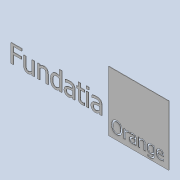
# Autodesk Inventor part: Orange
Saved by Autodesk Inventor 2020 (Build 240168000, 168)
## iProperties
Created: 2021-04-30
Part Number: Orange
Material: Generic
Document SubType Name: Modeling
Designer: Iulian Bors
Density: 1 g/cm^3
Appearance: Default
Author: Iulian Bors
Autodesk Inventor part; units mm, degrees
ref_plane "YZ Plane" through (0, 0, 0) normal (1, 0, 0) x (0, 1, 0)
ref_plane "XZ Plane" through (0, 0, 0) normal (0, 1, 0) x (-1, 0, 0)
ref_plane "XY Plane" through (0, 0, 0) normal (0, 0, 1) x (1, 0, 0)
sketch "Sketch1" plane through (0, 0, 0) normal (0, 0, 1) x (1, 0, 0)
  line L0 (-148.5, 210) -> (148.5, 210) construction
  line L1 (148.5, 210) -> (148.5, -210) construction
  line L2 (148.5, -210) -> (-148.5, -210) construction
  line L3 (-148.5, -210) -> (-148.5, 210) construction
  line L4 (22.4766, 60.7197) -> (122.4766, 60.7197)
  line L5 (122.4766, 60.7197) -> (122.4766, -39.2803)
  line L6 (122.4766, -39.2803) -> (22.4766, -39.2803)
  line L7 (22.4766, -39.2803) -> (22.4766, 60.7197)
  line L8 (26.6157, -0.7486) -> (40.1539, -0.7486) construction
  line L9 (40.1539, -0.7486) -> (40.1539, -4.7253) construction
  line L10 (40.1539, -4.7253) -> (26.6157, -4.7253) construction
  line L11 (26.6157, -4.7253) -> (26.6157, -0.7486) construction
  line L12 (-143.5348, 14.9841) -> (-38.9481, 14.9841) construction
  line L13 (-38.9481, 14.9841) -> (-38.9481, -7.7905) construction
  line L14 (-38.9481, -7.7905) -> (-143.5348, -7.7905) construction
  line L15 (-143.5348, -7.7905) -> (-143.5348, 14.9841) construction
  line L16 (-122.5543, 10.0975) -> (-136.5089, 10.0975)
  line L17 (-136.5089, 10.0975) -> (-136.5089, 1.6373)
  line L18 (-136.5089, 1.6373) -> (-123.1377, 1.6373)
  line L19 (-123.1377, 1.6373) -> (-123.1377, -1.9122)
  line L20 (-123.1377, -1.9122) -> (-136.5089, -1.9122)
  line L21 (-136.5089, -1.9122) -> (-136.5089, -16.353)
  line L22 (-136.5089, -16.353) -> (-140.4959, -16.353)
  line L23 (-140.4959, -16.353) -> (-140.4959, 13.647)
  line L24 (-140.4959, 13.647) -> (-122.5543, 13.647)
  line L25 (-122.5543, 13.647) -> (-122.5543, 10.0975)
  line L26 (-101.7682, -16.353) -> (-105.5608, -16.353)
  line L27 (-105.5608, -16.353) -> (-105.5608, -13.8733)
  spline S0 degree 2 poles (-105.5608, -13.8733) (-107.3112, -15.4049) (-110.4473, -16.9851) (-112.3922, -16.9851) knots 0 0 0 1 2 2 2
  spline S1 degree 2 poles (-112.3922, -16.9851) (-113.8509, -16.9851) (-116.4522, -16.0127) (-117.4003, -14.9673) knots 0 0 0 1 2 2 2
  spline S2 degree 2 poles (-117.4003, -14.9673) (-118.3728, -13.9219) (-119.4424, -10.7371) (-119.4424, -8.4519) knots 0 0 0 1 2 2 2
  line L28 (-119.4424, -8.4519) -> (-119.4424, 6.1591)
  line L29 (-119.4424, 6.1591) -> (-115.6499, 6.1591)
  line L30 (-115.6499, 6.1591) -> (-115.6499, -6.6772)
  spline S3 degree 2 poles (-115.6499, -6.6772) (-115.6499, -8.4762) (-115.3825, -10.8344) (-114.9206, -11.7096) knots 0 0 0 1 2 2 2
  spline S4 degree 2 poles (-114.9206, -11.7096) (-114.4587, -12.5848) (-112.8784, -13.3871) (-111.3954, -13.3871) knots 0 0 0 1 2 2 2
  spline S5 degree 2 poles (-111.3954, -13.3871) (-110.0097, -13.3871) (-106.8736, -11.8068) (-105.5608, -10.6642) knots 0 0 0 1 2 2 2
  line L31 (-105.5608, -10.6642) -> (-105.5608, 6.1591)
  line L32 (-105.5608, 6.1591) -> (-101.7682, 6.1591)
  line L33 (-101.7682, 6.1591) -> (-101.7682, -16.353)
  line L34 (-78.5997, -16.353) -> (-82.3922, -16.353)
  line L35 (-82.3922, -16.353) -> (-82.3922, -3.5167)
  spline S6 degree 2 poles (-82.3922, -3.5167) (-82.3922, -1.9608) (-82.6839, 0.7134) (-83.1215, 1.5157) knots 0 0 0 1 2 2 2
  spline S7 degree 2 poles (-83.1215, 1.5157) (-83.5835, 2.3666) (-85.2366, 3.1932) (-86.6467, 3.1932) knots 0 0 0 1 2 2 2
  spline S8 degree 2 poles (-86.6467, 3.1932) (-88.0567, 3.1932) (-91.047, 1.6859) (-92.4813, 0.4703) knots 0 0 0 1 2 2 2
  line L36 (-92.4813, 0.4703) -> (-92.4813, -16.353)
  line L37 (-92.4813, -16.353) -> (-96.2739, -16.353)
  line L38 (-96.2739, -16.353) -> (-96.2739, 6.1591)
  line L39 (-96.2739, 6.1591) -> (-92.4813, 6.1591)
  line L40 (-92.4813, 6.1591) -> (-92.4813, 3.6551)
  spline S9 degree 2 poles (-92.4813, 3.6551) (-90.7796, 5.1867) (-87.4976, 6.7912) (-85.6499, 6.7912) knots 0 0 0 1 2 2 2
  spline S10 degree 2 poles (-85.6499, 6.7912) (-82.3436, 6.7912) (-78.5997, 2.4152) (-78.5997, -1.742) knots 0 0 0 1 2 2 2
  line L41 (-78.5997, -1.742) -> (-78.5997, -16.353)
  line L42 (-55.9659, -16.353) -> (-59.7585, -16.353)
  line L43 (-59.7585, -16.353) -> (-59.7585, -14.0678)
  spline S11 degree 2 poles (-59.7585, -14.0678) (-60.6337, -14.7971) (-61.9222, -15.7696) (-62.7974, -16.1828) knots 0 0 0 1 2 2 2
  spline S12 degree 2 poles (-62.7974, -16.1828) (-63.5997, -16.5718) (-65.3258, -16.9851) (-66.4684, -16.9851) knots 0 0 0 1 2 2 2
  spline S13 degree 2 poles (-66.4684, -16.9851) (-68.316, -16.9851) (-71.4279, -15.4535) (-72.5219, -13.9705) knots 0 0 0 1 2 2 2
  spline S14 degree 2 poles (-72.5219, -13.9705) (-73.6159, -12.4875) (-74.8314, -8.1115) (-74.8314, -5.2671) knots 0 0 0 1 2 2 2
  spline S15 degree 2 poles (-74.8314, -5.2671) (-74.8314, -2.3012) (-73.2998, 2.0262) (-71.9627, 3.6551) knots 0 0 0 1 2 2 2
  spline S16 degree 2 poles (-71.9627, 3.6551) (-70.7228, 5.1138) (-67.2463, 6.7912) (-65.3258, 6.7912) knots 0 0 0 1 2 2 2
  spline S17 degree 2 poles (-65.3258, 6.7912) (-63.6483, 6.7912) (-61.1442, 6.0376) (-59.7585, 5.2596) knots 0 0 0 1 2 2 2
  line L44 (-59.7585, 5.2596) -> (-59.7585, 14.9841)
  line L45 (-59.7585, 14.9841) -> (-55.9659, 14.9841)
  line L46 (-55.9659, 14.9841) -> (-55.9659, -16.353)
  line L47 (-59.7585, -10.883) -> (-59.7585, 2.1235)
  spline S18 degree 2 poles (-59.7585, 2.1235) (-61.1685, 2.8042) (-63.4052, 3.3147) (-64.6937, 3.3147) knots 0 0 0 1 2 2 2
  spline S19 degree 2 poles (-64.6937, 3.3147) (-67.611, 3.3147) (-70.9173, -1.0613) (-70.9173, -5.1942) knots 0 0 0 1 2 2 2
  spline S20 degree 2 poles (-70.9173, -5.1942) (-70.9173, -9.1812) (-68.389, -13.3871) (-65.5932, -13.3871) knots 0 0 0 1 2 2 2
  spline S21 degree 2 poles (-65.5932, -13.3871) (-64.1102, -13.3871) (-61.0956, -12.0256) (-59.7585, -10.883) knots 0 0 0 1 2 2 2
  spline S22 degree 2 poles (-37.927, -13.9705) (-38.389, -14.3109) (-39.9449, -15.5264) (-40.6742, -15.8911) knots 0 0 0 1 2 2 2
  spline S23 degree 2 poles (-40.6742, -15.8911) (-41.671, -16.426) (-43.5429, -16.9851) (-45.2447, -16.9851) knots 0 0 0 1 2 2 2
  spline S24 degree 2 poles (-45.2447, -16.9851) (-46.6305, -16.9851) (-49.1345, -15.9397) (-50.0826, -14.9916) knots 0 0 0 1 2 2 2
  spline S25 degree 2 poles (-50.0826, -14.9916) (-50.9822, -14.0678) (-52.0762, -11.3449) (-52.0762, -9.8376) knots 0 0 0 1 2 2 2
  spline S26 degree 2 poles (-52.0762, -9.8376) (-52.0762, -7.5038) (-50.107, -4.1974) (-47.9676, -3.2493) knots 0 0 0 1 2 2 2
  spline S27 degree 2 poles (-47.9676, -3.2493) (-46.0713, -2.3741) (-40.9173, -1.7177) (-37.927, -1.5475) knots 0 0 0 1 2 2 2
  line L48 (-37.927, -1.5475) -> (-37.927, -0.8182)
  spline S28 degree 2 poles (-37.927, -0.8182) (-37.927, 0.4946) (-38.7293, 2.1235) (-39.4587, 2.5854) knots 0 0 0 1 2 2 2
  spline S29 degree 2 poles (-39.4587, 2.5854) (-40.188, 3.0473) (-42.2788, 3.339) (-43.3971, 3.339) knots 0 0 0 1 2 2 2
  spline S30 degree 2 poles (-43.3971, 3.339) (-44.7099, 3.339) (-48.2593, 2.5611) (-50.034, 1.8074) knots 0 0 0 1 2 2 2
  line L49 (-50.034, 1.8074) -> (-50.2528, 1.8074)
  line L50 (-50.2528, 1.8074) -> (-50.2528, 5.6729)
  spline S31 degree 2 poles (-50.2528, 5.6729) (-49.2074, 5.9646) (-45.2933, 6.694) (-43.3728, 6.694) knots 0 0 0 1 2 2 2
  spline S32 degree 2 poles (-43.3728, 6.694) (-41.0389, 6.694) (-37.8541, 5.9646) (-36.5899, 5.0165) knots 0 0 0 1 2 2 2
  spline S33 degree 2 poles (-36.5899, 5.0165) (-35.3501, 4.0927) (-34.1345, 1.151) (-34.1345, -0.964) knots 0 0 0 1 2 2 2
  line L51 (-34.1345, -0.964) -> (-34.1345, -16.353)
  line L52 (-34.1345, -16.353) -> (-37.927, -16.353)
  line L53 (-37.927, -16.353) -> (-37.927, -13.9705)
  line L54 (-37.927, -10.8101) -> (-37.927, -4.5621)
  spline S34 degree 2 poles (-37.927, -4.5621) (-39.2885, -4.6837) (-43.3971, -5.0969) (-44.6856, -5.4859) knots 0 0 0 1 2 2 2
  spline S35 degree 2 poles (-44.6856, -5.4859) (-46.1929, -5.9478) (-48.1621, -7.8684) (-48.1621, -9.5702) knots 0 0 0 1 2 2 2
  spline S36 degree 2 poles (-48.1621, -9.5702) (-48.1621, -11.5151) (-45.9741, -13.4843) (-43.8833, -13.4843) knots 0 0 0 1 2 2 2
  spline S37 degree 2 poles (-43.8833, -13.4843) (-42.1086, -13.4843) (-39.1912, -11.9527) (-37.927, -10.8101) knots 0 0 0 1 2 2 2
  spline S38 degree 2 poles (-22.0032, -16.7906) (-25.0907, -16.7906) (-28.5672, -13.2655) (-28.5672, -9.4486) knots 0 0 0 1 2 2 2
  line L55 (-28.5672, -9.4486) -> (-28.5672, 3.023)
  line L56 (-28.5672, 3.023) -> (-31.1199, 3.023)
  line L57 (-31.1199, 3.023) -> (-31.1199, 6.1591)
  line L58 (-31.1199, 6.1591) -> (-28.5672, 6.1591)
  line L59 (-28.5672, 6.1591) -> (-28.5672, 12.6259)
  line L60 (-28.5672, 12.6259) -> (-24.7747, 12.6259)
  line L61 (-24.7747, 12.6259) -> (-24.7747, 6.1591)
  line L62 (-24.7747, 6.1591) -> (-17.7974, 6.1591)
  line L63 (-17.7974, 6.1591) -> (-17.7974, 3.023)
  line L64 (-17.7974, 3.023) -> (-24.7747, 3.023)
  line L65 (-24.7747, 3.023) -> (-24.7747, -7.6982)
  spline S39 degree 2 poles (-24.7747, -7.6982) (-24.7747, -9.4) (-24.6531, -11.272) (-24.2399, -12.0743) knots 0 0 0 1 2 2 2
  spline S40 degree 2 poles (-24.2399, -12.0743) (-23.8995, -12.7793) (-22.3679, -13.4843) (-21.0551, -13.4843) knots 0 0 0 1 2 2 2
  spline S41 degree 2 poles (-21.0551, -13.4843) (-20.1313, -13.4843) (-18.4052, -12.9251) (-18.0162, -12.755) knots 0 0 0 1 2 2 2
  line L66 (-18.0162, -12.755) -> (-17.7974, -12.755)
  line L67 (-17.7974, -12.755) -> (-17.7974, -16.1585)
  spline S42 degree 2 poles (-17.7974, -16.1585) (-18.8671, -16.4503) (-21.0551, -16.7906) (-22.0032, -16.7906) knots 0 0 0 1 2 2 2
  line L68 (-11.1361, -16.353) -> (-14.9287, -16.353)
  line L69 (-14.9287, -16.353) -> (-14.9287, 6.1591)
  line L70 (-14.9287, 6.1591) -> (-11.1361, 6.1591)
  line L71 (-11.1361, 6.1591) -> (-11.1361, -16.353)
  line L72 (-10.8687, 9.9031) -> (-15.1718, 9.9031)
  line L73 (-15.1718, 9.9031) -> (-15.1718, 13.8415)
  line L74 (-15.1718, 13.8415) -> (-10.8687, 13.8415)
  line L75 (-10.8687, 13.8415) -> (-10.8687, 9.9031)
  spline S43 degree 2 poles (6.9757, -13.9705) (6.5138, -14.3109) (4.9579, -15.5264) (4.2285, -15.8911) knots 0 0 0 1 2 2 2
  spline S44 degree 2 poles (4.2285, -15.8911) (3.2318, -16.426) (1.3598, -16.9851) (-0.342, -16.9851) knots 0 0 0 1 2 2 2
  spline S45 degree 2 poles (-0.342, -16.9851) (-1.7277, -16.9851) (-4.2317, -15.9397) (-5.1799, -14.9916) knots 0 0 0 1 2 2 2
  spline S46 degree 2 poles (-5.1799, -14.9916) (-6.0794, -14.0678) (-7.1734, -11.3449) (-7.1734, -9.8376) knots 0 0 0 1 2 2 2
  spline S47 degree 2 poles (-7.1734, -9.8376) (-7.1734, -7.5038) (-5.2042, -4.1974) (-3.0648, -3.2493) knots 0 0 0 1 2 2 2
  spline S48 degree 2 poles (-3.0648, -3.2493) (-1.1685, -2.3741) (3.9854, -1.7177) (6.9757, -1.5475) knots 0 0 0 1 2 2 2
  line L76 (6.9757, -1.5475) -> (6.9757, -0.8182)
  spline S49 degree 2 poles (6.9757, -0.8182) (6.9757, 0.4946) (6.1734, 2.1235) (5.4441, 2.5854) knots 0 0 0 1 2 2 2
  spline S50 degree 2 poles (5.4441, 2.5854) (4.7148, 3.0473) (2.624, 3.339) (1.5057, 3.339) knots 0 0 0 1 2 2 2
  spline S51 degree 2 poles (1.5057, 3.339) (0.1929, 3.339) (-3.3565, 2.5611) (-5.1313, 1.8074) knots 0 0 0 1 2 2 2
  line L77 (-5.1313, 1.8074) -> (-5.3501, 1.8074)
  line L78 (-5.3501, 1.8074) -> (-5.3501, 5.6729)
  spline S52 degree 2 poles (-5.3501, 5.6729) (-4.3047, 5.9646) (-0.3906, 6.694) (1.53, 6.694) knots 0 0 0 1 2 2 2
  spline S53 degree 2 poles (1.53, 6.694) (3.8639, 6.694) (7.0486, 5.9646) (8.3128, 5.0165) knots 0 0 0 1 2 2 2
  spline S54 degree 2 poles (8.3128, 5.0165) (9.5527, 4.0927) (10.7683, 1.151) (10.7683, -0.964) knots 0 0 0 1 2 2 2
  line L79 (10.7683, -0.964) -> (10.7683, -16.353)
  line L80 (10.7683, -16.353) -> (6.9757, -16.353)
  line L81 (6.9757, -16.353) -> (6.9757, -13.9705)
  line L82 (6.9757, -10.8101) -> (6.9757, -4.5621)
  spline S55 degree 2 poles (6.9757, -4.5621) (5.6143, -4.6837) (1.5057, -5.0969) (0.2172, -5.4859) knots 0 0 0 1 2 2 2
  spline S56 degree 2 poles (0.2172, -5.4859) (-1.2901, -5.9478) (-3.2593, -7.8684) (-3.2593, -9.5702) knots 0 0 0 1 2 2 2
  spline S57 degree 2 poles (-3.2593, -9.5702) (-3.2593, -11.5151) (-1.0713, -13.4843) (1.0195, -13.4843) knots 0 0 0 1 2 2 2
  spline S58 degree 2 poles (1.0195, -13.4843) (2.7942, -13.4843) (5.7115, -11.9527) (6.9757, -10.8101) knots 0 0 0 1 2 2 2
  point P0 (0, 0)
  point P1 (0, 210)
  point P2 (-148.5, 0)
  dimension "d0" = 297
  dimension "d1" = 420
  dimension "d7" = 100
  dimension "d8" = 100
  constraints: 16 end point, 4 parallel, 2 horizontal, 2 midpoint, 2 perpendicular, 1 horizontal alignment, 1 vertical alignment, 4 other
  measures "d0" distance of L0.start L0.end
  measures "d1" distance of L2.end L0.start
  measures "d7" distance of L4.start L4.end
  measures "d8" distance of L6.end L4.start
extrude "Extrusion1" add sketch "Sketch1" along normal blind 0.8
sketch "Sketch2" plane through (0, 0, 0.8) normal (0, 0, 1) x (1, 0, 0)
  line L0 (26.5201, -10.6104) -> (115.3532, -10.6104) construction
  line L1 (115.3532, -10.6104) -> (115.3532, -36.7044) construction
  line L2 (115.3532, -36.7044) -> (26.5201, -36.7044) construction
  line L3 (26.5201, -36.7044) -> (26.5201, -10.6104) construction
  spline S0 degree 2 poles (42.6951, -13.3171) (43.8297, -14.6461) (45.0938, -18.5359) (45.0938, -21.0318) knots 0 0 0 1 2 2 2
  spline S1 degree 2 poles (45.0938, -21.0318) (45.0938, -23.463) (43.8621, -27.4014) (42.6951, -28.7304) knots 0 0 0 1 2 2 2
  spline S2 degree 2 poles (42.6951, -28.7304) (41.4634, -30.1242) (38.2057, -31.4532) (36.2446, -31.4532) knots 0 0 0 1 2 2 2
  spline S3 degree 2 poles (36.2446, -31.4532) (34.2186, -31.4532) (30.9771, -30.0756) (29.794, -28.7304) knots 0 0 0 1 2 2 2
  spline S4 degree 2 poles (29.794, -28.7304) (28.6433, -27.4014) (27.4115, -23.4954) (27.4115, -21.0318) knots 0 0 0 1 2 2 2
  spline S5 degree 2 poles (27.4115, -21.0318) (27.4115, -18.5197) (28.6595, -14.6947) (29.8102, -13.3171) knots 0 0 0 1 2 2 2
  spline S6 degree 2 poles (29.8102, -13.3171) (30.9771, -11.9881) (34.2348, -10.6104) (36.2446, -10.6104) knots 0 0 0 1 2 2 2
  spline S7 degree 2 poles (36.2446, -10.6104) (38.2867, -10.6104) (41.5606, -12.0367) (42.6951, -13.3171) knots 0 0 0 1 2 2 2
  spline S8 degree 2 poles (42.3224, -21.0318) (42.3224, -19.0545) (41.4634, -15.9913) (40.6854, -14.9865) knots 0 0 0 1 2 2 2
  spline S9 degree 2 poles (40.6854, -14.9865) (39.8912, -13.9492) (37.6546, -12.9119) (36.2608, -12.9119) knots 0 0 0 1 2 2 2
  spline S10 degree 2 poles (36.2608, -12.9119) (34.8183, -12.9119) (32.6465, -13.9168) (31.8199, -14.9865) knots 0 0 0 1 2 2 2
  spline S11 degree 2 poles (31.8199, -14.9865) (31.0258, -16.0075) (30.183, -19.0869) (30.183, -21.0318) knots 0 0 0 1 2 2 2
  spline S12 degree 2 poles (30.183, -21.0318) (30.183, -24.9702) (33.4893, -29.1518) (36.2608, -29.1518) knots 0 0 0 1 2 2 2
  spline S13 degree 2 poles (36.2608, -29.1518) (39.0323, -29.1518) (42.3224, -24.9702) (42.3224, -21.0318) knots 0 0 0 1 2 2 2
  line L4 (55.7746, -18.7304) -> (55.6449, -18.7304)
  spline S14 degree 2 poles (55.6449, -18.7304) (55.3532, -18.6493) (54.7211, -18.6169) (54.2835, -18.6169) knots 0 0 0 1 2 2 2
  spline S15 degree 2 poles (54.2835, -18.6169) (53.2624, -18.6169) (51.2527, -19.5083) (50.3451, -20.3835) knots 0 0 0 1 2 2 2
  line L5 (50.3451, -20.3835) -> (50.3451, -31.0318)
  line L6 (50.3451, -31.0318) -> (47.8167, -31.0318)
  line L7 (47.8167, -31.0318) -> (47.8167, -16.0237)
  line L8 (47.8167, -16.0237) -> (50.3451, -16.0237)
  line L9 (50.3451, -16.0237) -> (50.3451, -18.2604)
  spline S16 degree 2 poles (50.3451, -18.2604) (51.7227, -17.0286) (53.781, -16.0237) (54.7535, -16.0237) knots 0 0 0 1 2 2 2
  spline S17 degree 2 poles (54.7535, -16.0237) (55.1425, -16.0237) (55.5314, -16.0561) (55.7746, -16.1048) knots 0 0 0 1 2 2 2
  line L10 (55.7746, -16.1048) -> (55.7746, -18.7304)
  spline S18 degree 2 poles (66.0987, -29.4435) (65.7908, -29.6704) (64.7535, -30.4808) (64.2673, -30.7239) knots 0 0 0 1 2 2 2
  spline S19 degree 2 poles (64.2673, -30.7239) (63.6028, -31.0805) (62.3548, -31.4532) (61.2203, -31.4532) knots 0 0 0 1 2 2 2
  spline S20 degree 2 poles (61.2203, -31.4532) (60.2964, -31.4532) (58.6271, -30.7563) (57.995, -30.1242) knots 0 0 0 1 2 2 2
  spline S21 degree 2 poles (57.995, -30.1242) (57.3953, -29.5083) (56.666, -27.6931) (56.666, -26.6882) knots 0 0 0 1 2 2 2
  spline S22 degree 2 poles (56.666, -26.6882) (56.666, -25.1323) (57.9788, -22.9281) (59.405, -22.296) knots 0 0 0 1 2 2 2
  spline S23 degree 2 poles (59.405, -22.296) (60.6692, -21.7125) (64.1052, -21.2749) (66.0987, -21.1615) knots 0 0 0 1 2 2 2
  line L11 (66.0987, -21.1615) -> (66.0987, -20.6753)
  spline S24 degree 2 poles (66.0987, -20.6753) (66.0987, -19.8001) (65.5639, -18.7142) (65.0776, -18.4062) knots 0 0 0 1 2 2 2
  spline S25 degree 2 poles (65.0776, -18.4062) (64.5914, -18.0983) (63.1976, -17.9038) (62.452, -17.9038) knots 0 0 0 1 2 2 2
  spline S26 degree 2 poles (62.452, -17.9038) (61.5768, -17.9038) (59.2105, -18.4224) (58.0274, -18.9249) knots 0 0 0 1 2 2 2
  line L12 (58.0274, -18.9249) -> (57.8815, -18.9249)
  line L13 (57.8815, -18.9249) -> (57.8815, -16.3479)
  spline S27 degree 2 poles (57.8815, -16.3479) (58.5784, -16.1534) (61.1878, -15.6672) (62.4682, -15.6672) knots 0 0 0 1 2 2 2
  spline S28 degree 2 poles (62.4682, -15.6672) (64.0241, -15.6672) (66.1473, -16.1534) (66.9901, -16.7855) knots 0 0 0 1 2 2 2
  spline S29 degree 2 poles (66.9901, -16.7855) (67.8167, -17.4014) (68.6271, -19.3625) (68.6271, -20.7725) knots 0 0 0 1 2 2 2
  line L14 (68.6271, -20.7725) -> (68.6271, -31.0318)
  line L15 (68.6271, -31.0318) -> (66.0987, -31.0318)
  line L16 (66.0987, -31.0318) -> (66.0987, -29.4435)
  line L17 (66.0987, -27.3365) -> (66.0987, -23.1712)
  spline S30 degree 2 poles (66.0987, -23.1712) (65.1911, -23.2523) (62.452, -23.5278) (61.593, -23.7871) knots 0 0 0 1 2 2 2
  spline S31 degree 2 poles (61.593, -23.7871) (60.5882, -24.095) (59.2754, -25.3754) (59.2754, -26.51) knots 0 0 0 1 2 2 2
  spline S32 degree 2 poles (59.2754, -26.51) (59.2754, -27.8066) (60.734, -29.1194) (62.1279, -29.1194) knots 0 0 0 1 2 2 2
  spline S33 degree 2 poles (62.1279, -29.1194) (63.311, -29.1194) (65.2559, -28.0983) (66.0987, -27.3365) knots 0 0 0 1 2 2 2
  line L18 (83.9593, -31.0318) -> (81.431, -31.0318)
  line L19 (81.431, -31.0318) -> (81.431, -22.4743)
  spline S34 degree 2 poles (81.431, -22.4743) (81.431, -21.437) (81.2365, -19.6542) (80.9447, -19.1194) knots 0 0 0 1 2 2 2
  spline S35 degree 2 poles (80.9447, -19.1194) (80.6368, -18.5521) (79.5347, -18.001) (78.5946, -18.001) knots 0 0 0 1 2 2 2
  spline S36 degree 2 poles (78.5946, -18.001) (77.6546, -18.001) (75.6611, -19.0059) (74.7049, -19.8163) knots 0 0 0 1 2 2 2
  line L20 (74.7049, -19.8163) -> (74.7049, -31.0318)
  line L21 (74.7049, -31.0318) -> (72.1765, -31.0318)
  line L22 (72.1765, -31.0318) -> (72.1765, -16.0237)
  line L23 (72.1765, -16.0237) -> (74.7049, -16.0237)
  line L24 (74.7049, -16.0237) -> (74.7049, -17.6931)
  spline S37 degree 2 poles (74.7049, -17.6931) (75.8394, -16.672) (78.0274, -15.6023) (79.2592, -15.6023) knots 0 0 0 1 2 2 2
  spline S38 degree 2 poles (79.2592, -15.6023) (81.4634, -15.6023) (83.9593, -18.5197) (83.9593, -21.2912) knots 0 0 0 1 2 2 2
  line L25 (83.9593, -21.2912) -> (83.9593, -31.0318)
  spline S39 degree 2 poles (88.0436, -33.4305) (88.3029, -33.544) (89.2916, -33.9006) (89.9237, -34.0464) knots 0 0 0 1 2 2 2
  spline S40 degree 2 poles (89.9237, -34.0464) (90.6206, -34.2247) (91.8037, -34.4354) (92.5006, -34.4354) knots 0 0 0 1 2 2 2
  spline S41 degree 2 poles (92.5006, -34.4354) (93.6676, -34.4354) (95.2883, -33.8195) (95.7421, -33.2685) knots 0 0 0 1 2 2 2
  spline S42 degree 2 poles (95.7421, -33.2685) (96.1797, -32.7174) (96.5201, -31.2749) (96.5201, -30.3511) knots 0 0 0 1 2 2 2
  line L26 (96.5201, -30.3511) -> (96.5201, -29.0383)
  spline S43 degree 2 poles (96.5201, -29.0383) (95.499, -29.9297) (93.5379, -30.7725) (92.063, -30.7725) knots 0 0 0 1 2 2 2
  spline S44 degree 2 poles (92.063, -30.7725) (89.5023, -30.7725) (86.4715, -26.9638) (86.4715, -23.3819) knots 0 0 0 1 2 2 2
  spline S45 degree 2 poles (86.4715, -23.3819) (86.4715, -21.5181) (87.525, -18.6331) (88.4002, -17.6121) knots 0 0 0 1 2 2 2
  spline S46 degree 2 poles (88.4002, -17.6121) (89.2429, -16.6558) (91.5606, -15.6023) (92.7924, -15.6023) knots 0 0 0 1 2 2 2
  spline S47 degree 2 poles (92.7924, -15.6023) (93.9593, -15.6023) (95.6611, -16.1534) (96.5201, -16.6558) knots 0 0 0 1 2 2 2
  line L27 (96.5201, -16.6558) -> (96.666, -16.0237)
  line L28 (96.666, -16.0237) -> (99.0485, -16.0237)
  line L29 (99.0485, -16.0237) -> (99.0485, -29.3138)
  spline S48 degree 2 poles (99.0485, -29.3138) (99.0485, -33.1388) (95.7259, -36.7044) (92.3062, -36.7044) knots 0 0 0 1 2 2 2
  spline S49 degree 2 poles (92.3062, -36.7044) (91.204, -36.7044) (88.9026, -36.3479) (87.9139, -36.0561) knots 0 0 0 1 2 2 2
  line L30 (87.9139, -36.0561) -> (87.9139, -33.4305)
  line L31 (87.9139, -33.4305) -> (88.0436, -33.4305)
  line L32 (96.5201, -26.9638) -> (96.5201, -18.7142)
  spline S50 degree 2 poles (96.5201, -18.7142) (95.5801, -18.2604) (93.9917, -17.8714) (93.1976, -17.8714) knots 0 0 0 1 2 2 2
  spline S51 degree 2 poles (93.1976, -17.8714) (91.2851, -17.8714) (89.0809, -20.6915) (89.0809, -23.3333) knots 0 0 0 1 2 2 2
  spline S52 degree 2 poles (89.0809, -23.3333) (89.0809, -25.8292) (90.7502, -28.4386) (92.6303, -28.4386) knots 0 0 0 1 2 2 2
  spline S53 degree 2 poles (92.6303, -28.4386) (93.619, -28.4386) (95.6935, -27.6607) (96.5201, -26.9638) knots 0 0 0 1 2 2 2
  spline S54 degree 2 poles (109.2267, -31.3722) (105.6287, -31.3722) (101.6741, -27.3365) (101.6741, -23.6088) knots 0 0 0 1 2 2 2
  spline S55 degree 2 poles (101.6741, -23.6088) (101.6741, -19.9459) (105.5152, -15.6023) (108.6109, -15.6023) knots 0 0 0 1 2 2 2
  spline S56 degree 2 poles (108.6109, -15.6023) (110.0047, -15.6023) (112.1603, -16.4127) (112.9545, -17.2717) knots 0 0 0 1 2 2 2
  spline S57 degree 2 poles (112.9545, -17.2717) (113.7648, -18.1307) (114.6238, -20.6104) (114.6238, -22.4095) knots 0 0 0 1 2 2 2
  line L33 (114.6238, -22.4095) -> (114.6238, -23.7871)
  line L34 (114.6238, -23.7871) -> (104.2348, -23.7871)
  spline S58 degree 2 poles (104.2348, -23.7871) (104.2348, -26.3965) (106.8605, -29.168) (109.1943, -29.168) knots 0 0 0 1 2 2 2
  spline S59 degree 2 poles (109.1943, -29.168) (110.0209, -29.168) (111.6254, -28.7952) (112.2737, -28.5035) knots 0 0 0 1 2 2 2
  spline S60 degree 2 poles (112.2737, -28.5035) (112.9545, -28.1793) (113.8945, -27.6121) (114.2024, -27.3527) knots 0 0 0 1 2 2 2
  line L35 (114.2024, -27.3527) -> (114.3483, -27.3527)
  line L36 (114.3483, -27.3527) -> (114.3483, -30.108)
  spline S61 degree 2 poles (114.3483, -30.108) (113.9107, -30.2863) (112.5817, -30.8049) (112.063, -30.9508) knots 0 0 0 1 2 2 2
  spline S62 degree 2 poles (112.063, -30.9508) (111.3337, -31.1615) (110.1344, -31.3722) (109.2267, -31.3722) knots 0 0 0 1 2 2 2
  spline S63 degree 2 poles (112.1603, -21.8584) (112.1279, -20.8373) (111.7065, -19.3463) (111.3013, -18.8438) knots 0 0 0 1 2 2 2
  spline S64 degree 2 poles (111.3013, -18.8438) (110.8637, -18.2766) (109.4861, -17.6769) (108.465, -17.6769) knots 0 0 0 1 2 2 2
  spline S65 degree 2 poles (108.465, -17.6769) (107.4601, -17.6769) (106.0501, -18.2766) (105.4666, -18.86) knots 0 0 0 1 2 2 2
  spline S66 degree 2 poles (105.4666, -18.86) (104.8993, -19.4597) (104.3159, -20.9022) (104.2348, -21.8584) knots 0 0 0 1 2 2 2
  line L37 (104.2348, -21.8584) -> (112.1603, -21.8584)
  point P0 (0, 0)
  constraints: 2 other
extrude "Extrusion2" cut sketch "Sketch2" against normal through all
body "Solid1"
